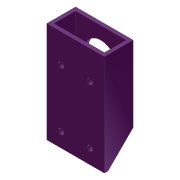
# Autodesk Inventor part: BearingMount
Saved by Autodesk Inventor 2012 (Build 160160000, 160)
## iProperties
Created: 2012-01-26
Part Number: BearingMount
Material: Aluminum-6061
Document SubType Name: Modeling
Designer: JesseK
Density: 2.71 g/cm^3
Mass: 88.5551 g
Surface Area: 220.576 cm^2
Volume: 32.6772 cm^3
Author: JesseK
Autodesk Inventor part; units mm, degrees
ref_plane "YZ Plane" through (0, 0, 0) normal (1, 0, 0) x (0, 1, 0)
ref_plane "XZ Plane" through (0, 0, 0) normal (0, 1, 0) x (-1, 0, 0)
ref_plane "XY Plane" through (0, 0, 0) normal (0, 0, 1) x (1, 0, 0)
sketch "Sketch1" plane through (0, 0, 0) normal (0, 0, 1) x (1, 0, 0)
  line L0 (0, 0) -> (50.8, 0)
  line L1 (50.8, 0) -> (50.8, 88.9)
  line L2 (50.8, 88.9) -> (0, 88.9)
  line L3 (0, 88.9) -> (0, 0)
  dimension "d0" = 50.8
  dimension "d1" = 88.9
  constraints: 8 end point, 2 parallel, 1 horizontal, 1 perpendicular
  measures "d0" distance of L0.start L0.end
  measures "d1" distance of L2.end L0.start
extrude "Extrusion1" add sketch "Sketch1" along normal blind 25.4
shell "Shell1" thickness 3.175 removed faces 2 at (33.8667, 88.9, 8.4667) at (16.9333, 0, 16.9333)
sketch "Sketch2" plane through (0, 0, 25.4) normal (0, 0, 1) x (1, 0, 0)
  line L0 (0, 0) -> (0, 88.9) projected
  line L1 (50.8, 0) -> (0, 0) projected
  line L2 (50.8, 88.9) -> (50.8, 0) projected
  line L3 (12.7, 63.5) -> (38.1, 63.5) construction
  line L4 (38.1, 63.5) -> (38.1, 12.7) construction
  line L5 (38.1, 12.7) -> (12.7, 12.7) construction
  line L6 (12.7, 12.7) -> (12.7, 63.5) construction
  line L7 (12.7, 63.5) -> (0, 63.5) construction
  line L8 (38.1, 63.5) -> (50.8, 63.5) construction
  line L9 (38.1, 12.7) -> (38.1, 0) construction
  circle A0 centre (12.7, 12.7) radius 2.4384
  circle A1 centre (38.1, 12.7) radius 2.4384
  circle A2 centre (38.1, 63.5) radius 2.4384
  circle A3 centre (12.7, 63.5) radius 2.4384
  dimension "d5" = 50.8
  dimension "d6" = 25.4
  dimension "d7" = 12.7
  dimension "d8" = 4.8768
  constraints: 14 end point, 4 centre point, 4 coincident, 3 equal radius, 3 horizontal, 3 point on line, 2 parallel, 1 collinear, 1 perpendicular, 1 vertical
  measures "d5" distance of L5.end L3.start
  measures "d6" distance of L3.start L3.end
  measures "d7" distance of L4.end L9.end
  measures "d8" diameter of A1
extrude "Extrusion2" cut sketch "Sketch2" against normal up to next
sketch "Sketch3" plane through (50.8, 0, 0) normal (1, 0, 0) x (0, 0, -1)
  line L0 (0, 0) -> (-25.4, 0) projected
  line L1 (0, 0) -> (0, 88.9) projected
  line L2 (-22.225, 0) -> (0, 22.225)
  line L3 (0, 22.225) -> (0, 0)
  line L4 (0, 0) -> (-22.225, 0)
  dimension "d11" = 22.225
  dimension "d12" = 22.225
  constraints: 6 end point, 2 point on line, 1 horizontal, 1 vertical
  measures "d11" distance of L0.start L2.start
  measures "d12" distance of L0.start L2.end
extrude "Extrusion3" cut sketch "Sketch3" against normal through all
sketch "Sketch5" plane through (0, 0, 0) normal (0, 0, -1) x (-1, 0, 0)
  line L0 (0, 88.9) -> (0, 22.225) projected
  circle A0 centre (-25.4, 63.5) radius 14.2875
  point P0 (0, 0)
  dimension "d19" = 63.5
  dimension "d20" = 28.575
  dimension "d21" = 25.4
  constraints: 1 centre point
  measures "d19" vertical distance of point (0, 0) A0.centre
  measures "d20" diameter of A0
  measures "d21" distance from line of L0 A0.centre
extrude "Extrusion5" cut sketch "Sketch5" against normal up to next
body "Solid1"
